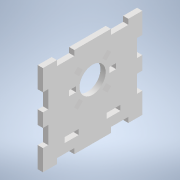
# Autodesk Inventor part: Frontal
Saved by Autodesk Inventor 2020.2 (Build 242310000, 310)
## iProperties
Created: 2020-03-18
Part Number: Frontal
Material: Generic
Document SubType Name: Modeling
Designer: ARQ SEVILLA R
Density: 1 g/cm^3
Appearance: Default
Author: ARQ SEVILLA R
Autodesk Inventor part; units mm, degrees
ref_plane "YZ Plane" through (0, 0, 0) normal (1, 0, 0) x (0, 1, 0)
ref_plane "XZ Plane" through (0, 0, 0) normal (0, 1, 0) x (-1, 0, 0)
ref_plane "XY Plane" through (0, 0, 0) normal (0, 0, 1) x (1, 0, 0)
sketch "Sketch1" plane through (0, 0, 0) normal (1, 0, 0) x (0, 1, 0)
  circle A0 centre (0, 0) radius 7.5
  line L0 (-31.75, -25.5) -> (-31.75, -20.5)
  line L1 (-31.75, -20.5) -> (-28.75, -20.5)
  line L2 (-28.75, -20.5) -> (-28.75, -10.5)
  line L3 (-28.75, -10.5) -> (-31.75, -10.5)
  line L4 (0, 0) -> (-31.75, 0) construction
  line L5 (-31.75, 20.5) -> (-28.75, 20.5)
  line L6 (-28.75, 20.5) -> (-28.75, 10.5)
  line L7 (-28.75, 10.5) -> (-31.75, 10.5)
  line L8 (-31.75, 25.5) -> (-31.75, 20.5)
  line L9 (-31.75, 10.5) -> (-31.75, -10.5)
  line L10 (-31.75, -20.5) -> (-31.75, -25.5)
  line L11 (20, 25.5) -> (20, 20.5)
  line L12 (20, 20.5) -> (17, 20.5)
  line L13 (17, 20.5) -> (17, 10.5)
  line L14 (17, 10.5) -> (20, 10.5)
  line L15 (20, -20.5) -> (17, -20.5)
  line L16 (17, -20.5) -> (17, -10.5)
  line L17 (17, -10.5) -> (20, -10.5)
  line L18 (20, 25.5) -> (20, 20.5)
  line L19 (20, 10.5) -> (20, -10.5)
  line L20 (20, -20.5) -> (20, -25.5)
  line L21 (20, 25.5) -> (20, 28.5)
  line L22 (-31.75, 28.5) -> (-31.75, 25.5)
  line L23 (-31.75, -25.5) -> (-31.75, -28.5)
  line L24 (20, -28.5) -> (20, -25.5)
  line L25 (-31.75, 28.5) -> (-19.75, 28.5)
  line L26 (-19.75, 28.5) -> (-19.75, 25.5)
  line L27 (-19.75, 25.5) -> (-9.75, 25.5)
  line L28 (-9.75, 25.5) -> (-9.75, 28.5)
  line L29 (-5.875, -28.5) -> (-5.875, 0) construction
  line L30 (8, 28.5) -> (8, 25.5)
  line L31 (8, 25.5) -> (-2, 25.5)
  line L32 (-2, 25.5) -> (-2, 28.5)
  line L33 (-19.75, -28.5) -> (-19.75, -25.5)
  line L34 (-19.75, -25.5) -> (-9.75, -25.5)
  line L35 (-9.75, -25.5) -> (-9.75, -28.5)
  line L36 (8, -25.5) -> (-2, -25.5)
  line L37 (8, -28.5) -> (8, -25.5)
  line L38 (-2, -25.5) -> (-2, -28.5)
  line L39 (-19.75, 28.5) -> (-31.75, 28.5)
  line L40 (20, 28.5) -> (8, 28.5)
  line L41 (-2, 28.5) -> (-9.75, 28.5)
  line L42 (-31.75, -28.5) -> (-19.75, -28.5)
  line L43 (-9.75, -28.5) -> (-2, -28.5)
  line L44 (8, -28.5) -> (20, -28.5)
  line L45 (-31.75, -28.5) -> (-19.75, -28.5)
  line L46 (-9.75, -28.5) -> (-5.875, -28.5)
  line L47 (-28.75, 20.5) -> (-23.5, 20.5) construction
  line L48 (-23.5, 20.5) -> (-23.5, -28.5) construction
  line L49 (-23.5, 0) -> (-23.5, -8) construction
  line L50 (-23.5, -8) -> (-20.5, -8)
  line L51 (-20.5, -8) -> (-20.5, -16)
  line L52 (-20.5, -16) -> (-23.5, -16)
  line L53 (-23.5, -8) -> (-23.5, -16)
  line L54 (-23.5, -20.5) -> (-23.5, 28.5) construction
  line L55 (-23.5, 0) -> (-23.5, 8) construction
  line L56 (-23.5, 8) -> (-20.5, 8)
  line L57 (-20.5, 8) -> (-20.5, 16)
  line L58 (-20.5, 16) -> (-23.5, 16)
  line L59 (-23.5, 8) -> (-23.5, 16)
  line L60 (0, -7.5) -> (0, -9.5) construction
  line L61 (0, -9.5) -> (1.5, -9.5)
  line L62 (1.5, -9.5) -> (1.5, -13.5)
  line L63 (1.5, -13.5) -> (-1.5, -13.5)
  line L64 (-1.5, -13.5) -> (-1.5, -9.5)
  line L65 (-1.5, -9.5) -> (0, -9.5)
  line L66 (0, 9.5) -> (1.5, 9.5)
  line L67 (1.5, 9.5) -> (1.5, 13.5)
  line L68 (1.5, 13.5) -> (-1.5, 13.5)
  line L69 (-1.5, 13.5) -> (-1.5, 9.5)
  line L70 (-1.5, 9.5) -> (0, 9.5)
  line L71 (7.5, 0) -> (9.5, 0) construction
  line L72 (9.5, 0) -> (9.5, -1.5)
  line L73 (9.5, -1.5) -> (13.5, -1.5)
  line L74 (13.5, -1.5) -> (13.5, 1.5)
  line L75 (13.5, 1.5) -> (9.5, 1.5)
  line L76 (9.5, 1.5) -> (9.5, 0)
  line L77 (-7.5, 0) -> (-9.5, 0) construction
  line L78 (-9.5, 0) -> (-9.5, -1.5)
  line L79 (-9.5, -1.5) -> (-13.5, -1.5)
  line L80 (-13.5, -1.5) -> (-13.5, 1.5)
  line L81 (-13.5, 1.5) -> (-9.5, 1.5)
  line L82 (-9.5, 1.5) -> (-9.5, 0)
  dimension "d0" = 15
  dimension "d3" = 51
  dimension "d7" = 5
  dimension "d8" = 3
  dimension "d9" = 10
  dimension "d10" = 3
  dimension "d11" = 51.75
  dimension "d12" = 3
  dimension "d13" = 3
  dimension "d14" = 12
  dimension "d15" = 3
  dimension "d16" = 10
  dimension "d17" = 25.875
  dimension "d18" = 5.25
  dimension "d19" = 8
  dimension "d20" = 3
  dimension "d21" = 8
  dimension "d22" = 2
  dimension "d23" = 1.5
  dimension "d24" = 4
  dimension "d25" = 3
  dimension "d26" = 2
  dimension "d27" = 1.5
  dimension "d28" = 4
  dimension "d29" = 3
  constraints: 166 end point, 42 perpendicular, 37 symmetric about line, 16 point on line, 3 vertical, 2 midpoint, 2 point on circle, 1 centre point, 1 coincident, 1 collinear, 1 horizontal
  measures "d0" diameter of A0
  measures "d3" distance of L11.start L20.end
  measures "d7" distance of L0.start L0.end
  measures "d8" distance of L0.end L1.end
  measures "d9" distance of L1.end L2.end
  measures "d10" distance of L11.end L12.end
  measures "d11" distance of L0.start L20.end
  measures "d12" distance of L11.start L21.end
  measures "d13" distance of L0.start L23.end
  measures "d14" distance of L22.start L25.end
  measures "d15" distance of L25.end L26.end
  measures "d16" distance of L26.end L27.end
  measures "d17" distance of L23.end L29.start
  measures "d18" distance of L6.start L47.end
  measures "d19" distance of L49.start L49.end
  measures "d20" distance of L49.end L50.end
  measures "d21" distance of L50.end L51.end
  measures "d22" distance of L60.start L60.end
  measures "d23" distance of L60.end L61.end
  measures "d24" distance of L61.end L62.end
  measures "d25" distance of L62.end L63.end
  measures "d26" distance of L71.start L71.end
  measures "d27" distance of L71.end L72.end
  measures "d28" distance of L72.end L73.end
  measures "d29" distance of L73.end L74.end
extrude "Extrusion1" add sketch "Sketch1" along normal blind 3
sketch "Sketch4" plane through (3, 0, 0) normal (1, 0, 0) x (0, 0, -1)
  line L0 (1.5, 9.5) -> (-1.5, 9.5) projected
  line L1 (-1.5, 9.5) -> (1.5, 9.5)
  line L2 (1.5, 13.5) -> (1.5, 9.5) projected
  line L3 (1.5, 9.5) -> (1.5, 13.5)
  line L4 (-1.5, 13.5) -> (1.5, 13.5) projected
  line L5 (1.5, 13.5) -> (-1.5, 13.5)
  line L6 (-1.5, 9.5) -> (-1.5, 13.5) projected
  line L7 (-1.5, 13.5) -> (-1.5, 9.5)
  line L8 (-1.5, -9.5) -> (1.5, -9.5) projected
  line L9 (-1.5, -9.5) -> (1.5, -9.5)
  line L10 (1.5, -9.5) -> (1.5, -13.5) projected
  line L11 (1.5, -9.5) -> (1.5, -13.5)
  line L12 (1.5, -13.5) -> (-1.5, -13.5) projected
  line L13 (1.5, -13.5) -> (-1.5, -13.5)
  line L14 (-1.5, -13.5) -> (-1.5, -9.5) projected
  line L15 (-1.5, -13.5) -> (-1.5, -9.5)
  point P0 (0, 0)
  constraints: 16 end point, 6 collinear, 1 horizontal, 1 perpendicular
extrude "Extrusion3" add sketch "Sketch4" against normal up to surface (3 mm away)
sketch "Sketch5" plane through (3, 0, 0) normal (1, 0, 0) x (0, 0, -1)
  line L0 (-9.5, -1.5) -> (-13.5, -1.5) projected
  line L1 (-13.5, -1.5) -> (-13.5, 1.5) projected
  line L2 (-13.5, 1.5) -> (-9.5, 1.5) projected
  line L3 (-9.5, 1.5) -> (-9.5, -1.5) projected
  line L4 (-9.5, -1.5) -> (-13.5, -1.5) projected
  line L5 (-13.5, -1.5) -> (-13.5, 1.5) projected
  line L6 (-13.5, -1.5) -> (-13.5, 1.5)
  line L7 (-13.5, 1.5) -> (-9.5, 1.5) projected
  line L8 (-13.5, 1.5) -> (-9.5, 1.5)
  line L9 (-9.5, 1.5) -> (-9.5, -1.5)
  line L10 (-13.5, -1.5) -> (-9.5, -1.5)
  line L11 (0, 0) -> (0, 8.8912) construction
  line L12 (-8.4853, -10.6066) -> (-10.6066, -8.4853)
  line L13 (-10.6066, -8.4853) -> (-7.7782, -5.6569)
  line L14 (-7.7782, -5.6569) -> (-5.6569, -7.7782)
  line L15 (-8.4853, -10.6066) -> (-5.6569, -7.7782)
  line L16 (8.4853, -10.6066) -> (5.6569, -7.7782)
  line L17 (10.6066, -8.4853) -> (8.4853, -10.6066)
  line L18 (10.6066, -8.4853) -> (7.7782, -5.6569)
  line L19 (5.6569, -7.7782) -> (7.7782, -5.6569)
  line L20 (0, 0) -> (-7.7782, 0) construction
  line L21 (-10.6066, 8.4853) -> (-7.7782, 5.6569)
  line L22 (-8.4853, 10.6066) -> (-10.6066, 8.4853)
  line L23 (-8.4853, 10.6066) -> (-5.6569, 7.7782)
  line L24 (-7.7782, 5.6569) -> (-5.6569, 7.7782)
  line L25 (10.6066, 8.4853) -> (7.7782, 5.6569)
  line L26 (5.6569, 7.7782) -> (7.7782, 5.6569)
  line L27 (8.4853, 10.6066) -> (5.6569, 7.7782)
  line L28 (10.6066, 8.4853) -> (8.4853, 10.6066)
  constraints: 44 end point, 9 perpendicular, 8 symmetric about line, 1 collinear, 1 horizontal, 1 vertical
extrude "Extrusion4" cut sketch "Sketch5" against normal up to surface (3 mm away) contours L12 L13 L14 L15 | L16 L19 L18 L17 | L22 L23 L24 L21 | L25 L26 L27 L28
ref_plane "Work Plane1" through (-17.5, 0, 0) normal (1, 0, 0) x (0, 0, -1)
sketch "Sketch6" plane through (-17.5, 0, 0) normal (1, 0, 0) x (0, 0, -1)
  line L0 (8.4853, -10.6066) -> (5.6569, -7.7782) projected
  line L1 (5.6569, -7.7782) -> (7.7782, -5.6569) projected
  line L2 (7.7782, -5.6569) -> (10.6066, -8.4853) projected
  line L3 (10.6066, -8.4853) -> (8.4853, -10.6066) projected
  line L4 (-5.6569, 7.7782) -> (-7.7782, 5.6569) projected
  line L5 (-7.7782, 5.6569) -> (-10.6066, 8.4853) projected
  line L6 (-10.6066, 8.4853) -> (-8.4853, 10.6066) projected
  line L7 (-8.4853, 10.6066) -> (-5.6569, 7.7782) projected
  line L8 (10.6066, 8.4853) -> (7.7782, 5.6569) projected
  line L9 (7.7782, 5.6569) -> (5.6569, 7.7782) projected
  line L10 (5.6569, 7.7782) -> (8.4853, 10.6066) projected
  line L11 (8.4853, 10.6066) -> (10.6066, 8.4853) projected
  line L12 (-7.7782, -5.6569) -> (-5.6569, -7.7782) projected
  line L13 (-5.6569, -7.7782) -> (-8.4853, -10.6066) projected
  line L14 (-8.4853, -10.6066) -> (-10.6066, -8.4853) projected
  line L15 (-10.6066, -8.4853) -> (-7.7782, -5.6569) projected
  line L16 (-25.5, -2) -> (-28.5, -2) projected
  line L17 (-28.5, -2) -> (-28.5, -9.75) projected
  line L18 (-28.5, -9.75) -> (-25.5, -9.75) projected
  line L19 (-25.5, -9.75) -> (-25.5, -19.75) projected
  line L20 (-25.5, -19.75) -> (-28.5, -19.75) projected
  line L21 (-28.5, -19.75) -> (-28.5, -31.75) projected
  line L22 (-28.5, -31.75) -> (-20.5, -31.75) projected
  line L23 (-20.5, -31.75) -> (-20.5, -28.75) projected
  line L24 (-20.5, -28.75) -> (-10.5, -28.75) projected
  line L25 (-10.5, -28.75) -> (-10.5, -31.75) projected
  line L26 (-10.5, -31.75) -> (10.5, -31.75) projected
  line L27 (10.5, -31.75) -> (10.5, -28.75) projected
  line L28 (10.5, -28.75) -> (20.5, -28.75) projected
  line L29 (20.5, -28.75) -> (20.5, -31.75) projected
  line L30 (20.5, -31.75) -> (28.5, -31.75) projected
  line L31 (28.5, -31.75) -> (28.5, -19.75) projected
  line L32 (28.5, -19.75) -> (25.5, -19.75) projected
  line L33 (25.5, -19.75) -> (25.5, -9.75) projected
  line L34 (25.5, -9.75) -> (28.5, -9.75) projected
  line L35 (28.5, -9.75) -> (28.5, -2) projected
  line L36 (28.5, -2) -> (25.5, -2) projected
  line L37 (25.5, -2) -> (25.5, 8) projected
  line L38 (25.5, 8) -> (28.5, 8) projected
  line L39 (28.5, 8) -> (28.5, 20) projected
  line L40 (28.5, 20) -> (20.5, 20) projected
  line L41 (20.5, 20) -> (20.5, 17) projected
  line L42 (20.5, 17) -> (10.5, 17) projected
  line L43 (10.5, 17) -> (10.5, 20) projected
  line L44 (10.5, 20) -> (-10.5, 20) projected
  line L45 (-10.5, 20) -> (-10.5, 17) projected
  line L46 (-10.5, 17) -> (-20.5, 17) projected
  line L47 (-20.5, 17) -> (-20.5, 20) projected
  line L48 (-20.5, 20) -> (-28.5, 20) projected
  line L49 (-28.5, 20) -> (-28.5, 8) projected
  line L50 (-28.5, 8) -> (-25.5, 8) projected
  line L51 (-25.5, 8) -> (-25.5, -2) projected
  circle A0 centre (0, 0) radius 7.5 projected
  line L52 (16, -20.5) -> (16, -23.5) projected
  line L53 (16, -23.5) -> (8, -23.5) projected
  line L54 (8, -23.5) -> (8, -20.5) projected
  line L55 (8, -20.5) -> (16, -20.5) projected
  line L56 (-8, -23.5) -> (-16, -23.5) projected
  line L57 (-16, -23.5) -> (-16, -20.5) projected
  line L58 (-16, -20.5) -> (-8, -20.5) projected
  line L59 (-8, -20.5) -> (-8, -23.5) projected
  line L60 (13.5, 1.5) -> (13.5, -1.5) projected
  line L61 (13.5, -1.5) -> (9.5, -1.5) projected
  line L62 (9.5, -1.5) -> (9.5, 1.5) projected
  line L63 (9.5, 1.5) -> (13.5, 1.5) projected
  line L64 (-9.5, 1.5) -> (-9.5, -1.5) projected
  line L65 (-9.5, -1.5) -> (-13.5, -1.5) projected
  line L66 (-13.5, -1.5) -> (-13.5, 1.5) projected
  line L67 (-13.5, 1.5) -> (-9.5, 1.5) projected
  circle A1 centre (0, 0) radius 14.5
  dimension "d40" = 29
  constraints: 1 centre point, 1 coincident
  measures "d40" diameter of A1
sketch "Sketch7" plane through (3, 0, 0) normal (1, 0, 0) x (0, 0, -1)
  line L0 (-13.5, -1.5) -> (-13.5, 1.5) projected
  line L1 (-9.5, 1.5) -> (-9.5, -1.5) projected
  line L2 (-13.5, -1.5) -> (-9.5, -1.5)
  line L3 (-9.5, -1.5) -> (-9.5, 1.5)
  line L4 (-9.5, 1.5) -> (-13.5, 1.5)
  line L5 (-13.5, 1.5) -> (-13.5, -1.5)
  line L6 (13.5, -1.5) -> (9.5, -1.5) projected
  line L7 (13.5, 1.5) -> (13.5, -1.5) projected
  line L8 (9.5, -1.5) -> (13.5, -1.5)
  line L9 (13.5, -1.5) -> (13.5, 1.5)
  line L10 (13.5, 1.5) -> (9.5, 1.5)
  line L11 (9.5, 1.5) -> (9.5, -1.5)
  point P0 (0, 0)
  constraints: 16 end point, 4 parallel, 2 horizontal, 2 perpendicular
extrude "Extrusion5" add sketch "Sketch7" against normal up to surface (3 mm away)
sketch "Sketch8" plane through (3, 0, 0) normal (1, 0, 0) x (0, 0, -1)
  line L0 (-8.4853, -10.6066) -> (-5.6569, -7.7782) projected
  line L1 (-8.4853, -10.6066) -> (-5.6569, -7.7782)
  line L2 (-5.6569, -7.7782) -> (-7.7782, -5.6569) projected
  line L3 (-5.6569, -7.7782) -> (-7.7782, -5.6569)
  line L4 (-7.7782, -5.6569) -> (-10.6066, -8.4853)
  line L5 (-10.6066, -8.4853) -> (-8.4853, -10.6066) projected
  line L6 (-10.6066, -8.4853) -> (-8.4853, -10.6066)
  line L7 (1.5, -13.5) -> (1.5, -9.5)
  line L8 (1.5, -9.5) -> (-1.5, -9.5)
  line L9 (-1.5, -9.5) -> (-1.5, -13.5)
  line L10 (-1.5, -13.5) -> (1.5, -13.5)
  point P0 (0, 0)
  constraints: 16 end point, 3 collinear, 2 perpendicular
extrude "Extrusion6" cut sketch "Sketch8" against normal up to surface (3 mm away) contours L10 L9 L8 L7
body "Solid1"
